Autodesk Fusion 360 part; units mm, degrees
(part 2 of 2)
sketch "Sketch3 (4)" plane through (0, 0, 356.35) normal (0, 0, 1) x (-1, 0, 0) in component "Roof"
  circle A0 centre (0, -130.225) radius 14.5
  line L0 (19.05, -257.175) -> (19.05, -263.525)
  line L1 (19.05, -263.525) -> (-19.05, -263.525)
  line L2 (-19.05, -263.525) -> (-19.05, -257.175)
  line L3 (-19.05, -257.175) -> (19.05, -257.175)
  line L4 (-126.35, -111.125) -> (-120, -111.125)
  line L5 (-120, -111.125) -> (-120, -149.225)
  line L6 (-120, -149.225) -> (-126.35, -149.225)
  line L7 (-126.35, -149.225) -> (-126.35, -111.125)
  line L8 (-19.05, 3.075) -> (19.05, 3.075)
  line L9 (19.05, 3.075) -> (19.05, -3.275)
  line L10 (19.05, -3.275) -> (-19.05, -3.275)
  line L11 (-19.05, -3.275) -> (-19.05, 3.075)
  line L12 (120, -111.1333) -> (126.35, -111.1333)
  line L13 (126.35, -111.1333) -> (126.35, -149.2333)
  line L14 (126.35, -149.2333) -> (120, -149.2333)
  line L15 (120, -149.2333) -> (120, -111.1333)
  line L16 (136.35, 13.325) -> (-136.35, 13.325)
  line L17 (-136.35, 13.325) -> (-136.35, -273.775)
  line L18 (-136.35, -273.775) -> (136.35, -273.775)
  line L19 (136.35, -273.775) -> (136.35, 13.325)
  circle A1 centre (0, -175.225) radius 10.5
  circle A2 centre (-14.1421, -189.3671) radius 6
  circle A3 centre (-14.1421, -161.0829) radius 6
  circle A4 centre (14.1421, -161.0829) radius 6
  circle A5 centre (14.1421, -189.3671) radius 6
  dimension "d238" = 21
  dimension "d239" = 12
  dimension "d240" = 12
  dimension "d241" = 12
  dimension "d242" = 12
  dimension "d243" = 20
  dimension "d244" = 20
  dimension "d245" = 20
  dimension "d246" = 20
  dimension "d247" = 45
  measures "d238" diameter of A1
  measures "d239" diameter of A2
  measures "d240" diameter of A3
  measures "d241" diameter of A4
  measures "d242" diameter of A5
  measures "d243" distance of A1.centre A4.centre
  measures "d244" distance of A1.centre A3.centre
  measures "d245" distance of A1.centre A2.centre
  measures "d246" distance of A1.centre A5.centre
  measures "d247" distance of A0.centre A1.centre
extrude "Extrude3'''" cut sketch "Sketch3 (4)" against normal blind 10 contours A1 | A2 | A3 | A4 | A5 bodies 9 in component "Roof"
sketch "Sketch4 (3)" plane through (0, 0, 356.35) normal (0, 0, 1) x (-1, 0, 0) in component "Roof"
  circle A0 centre (14.1421, -161.0829) radius 6
  circle A1 centre (0, -175.225) radius 10.5
  circle A2 centre (-14.1421, -161.0829) radius 6
  circle A3 centre (14.1421, -189.3671) radius 6
  circle A4 centre (-14.1421, -189.3671) radius 6
  circle A5 centre (0, -130.225) radius 14.5
  line L0 (19.05, -257.175) -> (19.05, -263.525)
  line L1 (19.05, -263.525) -> (-19.05, -263.525)
  line L2 (-19.05, -263.525) -> (-19.05, -257.175)
  line L3 (-19.05, -257.175) -> (19.05, -257.175)
  line L4 (-126.35, -111.125) -> (-120, -111.125)
  line L5 (-120, -111.125) -> (-120, -149.225)
  line L6 (-120, -149.225) -> (-126.35, -149.225)
  line L7 (-126.35, -149.225) -> (-126.35, -111.125)
  line L8 (-19.05, 3.075) -> (19.05, 3.075)
  line L9 (19.05, 3.075) -> (19.05, -3.275)
  line L10 (19.05, -3.275) -> (-19.05, -3.275)
  line L11 (-19.05, -3.275) -> (-19.05, 3.075)
  line L12 (120, -111.1333) -> (126.35, -111.1333)
  line L13 (126.35, -111.1333) -> (126.35, -149.2333)
  line L14 (126.35, -149.2333) -> (120, -149.2333)
  line L15 (120, -149.2333) -> (120, -111.1333)
  line L16 (136.35, 13.325) -> (-136.35, 13.325)
  line L17 (-136.35, 13.325) -> (-136.35, -273.775)
  line L18 (-136.35, -273.775) -> (136.35, -273.775)
  line L19 (136.35, -273.775) -> (136.35, 13.325)
  line L20 (-10.3078, -177.225) -> (-136.35, -177.225)
  line L21 (-136.35, -177.225) -> (-136.35, -173.225)
  line L22 (-136.35, -173.225) -> (-10.3078, -173.225)
  line L23 (-10.3078, -173.225) -> (-10.3078, -177.225)
  dimension "d250" = 2
  dimension "d251" = 2
  constraint horizontal L20
  constraint vertical L21
  constraint horizontal L22
  constraint vertical L23
  constraint coincident L17 L21.end
  constraint coincident A1 L20.start
  measures "d250" distance of A1.centre L20
  measures "d251" distance of A1.centre L22
extrude "Extrude4'''" cut sketch "Sketch4 (3)" against normal blind 6.35 contours A1 L17 L20 L21 L22 bodies 9 in component "Roof"
sketch "Sketch2 (5)" plane through (-126.35, 0, 0) normal (-1, 0, 0) x (0, -1, 0) in component "Left Wall"
  circle A0 centre (-130.175, 177.8) radius 31.75
  line L0 (-149.225, 25.4) -> (-149.225, 31.75)
  line L1 (-149.225, 31.75) -> (-111.125, 31.75)
  line L2 (-111.125, 31.75) -> (-111.125, 25.4)
  line L3 (-111.125, 25.4) -> (-149.225, 25.4)
  circle A1 centre (-183.675, 290) radius 5
  circle A2 centre (-98.075, 290) radius 5
  circle A3 centre (-33.875, 310) radius 5
  circle A4 centre (-119.475, 310) radius 5
  circle A5 centre (-205.075, 310) radius 5
  circle A6 centre (-183.675, 330) radius 5
  circle A7 centre (-98.075, 330) radius 5
  circle A8 centre (-33.875, 330) radius 5
  circle A9 centre (-119.475, 330) radius 5
  circle A10 centre (-205.075, 330) radius 5
  circle A11 centre (-183.675, 310) radius 5
  circle A12 centre (-98.075, 310) radius 5
  circle A13 centre (-33.875, 290) radius 5
  circle A14 centre (-119.475, 290) radius 5
  circle A15 centre (-205.075, 290) radius 5
  circle A16 centre (-162.275, 290) radius 5
  circle A17 centre (-76.675, 290) radius 5
  circle A18 centre (-55.275, 310) radius 5
  circle A19 centre (-162.275, 310) radius 5
  circle A20 centre (-226.4722, 310.344) radius 5
  circle A21 centre (-162.275, 330) radius 5
  circle A22 centre (-76.675, 330) radius 5
  circle A23 centre (-55.275, 330) radius 5
  circle A24 centre (-140.875, 330) radius 5
  circle A25 centre (-226.475, 330) radius 5
  circle A26 centre (-140.875, 310) radius 5
  circle A27 centre (-76.675, 310) radius 5
  circle A28 centre (-55.275, 290) radius 5
  circle A29 centre (-140.875, 290) radius 5
  circle A30 centre (-226.475, 290) radius 5
  line L4 (-3.175, 330.95) -> (-3.175, 350)
  line L5 (-3.175, 350) -> (-111.125, 350)
  line L6 (-111.125, 350) -> (-111.125, 370)
  line L7 (-111.125, 370) -> (-149.225, 370)
  line L8 (-149.225, 370) -> (-149.225, 350)
  line L9 (-149.225, 350) -> (-257.175, 350)
  line L10 (-257.175, 350) -> (-257.175, 330.95)
  line L11 (-257.175, 330.95) -> (-263.525, 330.95)
  line L12 (-263.525, 330.95) -> (-263.525, 350)
  line L13 (-263.525, 350) -> (-273.675, 350)
  line L14 (-273.675, 350) -> (-273.675, 311.9)
  line L15 (-273.675, 311.9) -> (-257.175, 311.9)
  line L16 (-257.175, 311.9) -> (-257.175, 0)
  line L17 (-257.175, 0) -> (-3.175, 0)
  line L18 (-3.175, 0) -> (-3.175, 311.9)
  line L19 (-3.175, 311.9) -> (13.325, 311.9)
  line L20 (13.325, 311.9) -> (13.325, 350)
  line L21 (13.325, 350) -> (3.175, 350)
  line L22 (3.175, 350) -> (3.175, 330.95)
  line L23 (3.175, 330.95) -> (-3.175, 330.95)
  line L24 (-140.175, 55.75) -> (-120.175, 55.75)
  line L25 (-120.175, 55.75) -> (-120.175, 43.75)
  line L26 (-120.175, 43.75) -> (-140.175, 43.75)
  line L27 (-140.175, 43.75) -> (-140.175, 55.75)
  dimension "d254" = 20
  dimension "d255" = 12
  dimension "d256" = 117
  dimension "d265" = 12
  constraint horizontal L24
  constraint vertical L25
  constraint horizontal L26
  constraint vertical L27
  measures "d254" distance of L24.start L24.end
  measures "d255" distance of L24.end L25.end
  measures "d256" distance of L18 L25
  measures "d265" distance of L1 L26
extrude "Extrude2'''''" cut sketch "Sketch2 (5)" against normal blind 20 contours L24 L25 L26 L27 bodies 6 in component "Left Wall"
sketch "Sketch1 (7)" plane through (0, -3.175, 0) normal (0, -1, 0) x (1, 0, 0) in component "Front Wall"
  line L0 (19.05, 31.75) -> (19.05, 25.4)
  line L1 (19.05, 25.4) -> (-19.05, 25.4)
  line L2 (-19.05, 25.4) -> (-19.05, 31.75)
  line L3 (-19.05, 31.75) -> (19.05, 31.75)
  circle A0 centre (50, 290) radius 5
  circle A1 centre (-30, 290) radius 5
  circle A2 centre (-90, 310) radius 5
  circle A3 centre (-10, 310) radius 5
  circle A4 centre (70, 310) radius 5
  circle A5 centre (50, 330) radius 5
  circle A6 centre (-30, 330) radius 5
  circle A7 centre (-90, 330) radius 5
  circle A8 centre (-10, 330) radius 5
  circle A9 centre (70, 330) radius 5
  circle A10 centre (50, 310) radius 5
  circle A11 centre (-30, 310) radius 5
  circle A12 centre (-90, 290) radius 5
  circle A13 centre (-10, 290) radius 5
  circle A14 centre (70, 290) radius 5
  circle A15 centre (30, 290) radius 5
  circle A16 centre (-50, 290) radius 5
  circle A17 centre (-70, 310) radius 5
  circle A18 centre (10, 310) radius 5
  circle A19 centre (90, 310) radius 5
  circle A20 centre (30, 330) radius 5
  circle A21 centre (-50, 330) radius 5
  circle A22 centre (-70, 330) radius 5
  circle A23 centre (10, 330) radius 5
  circle A24 centre (90, 330) radius 5
  circle A25 centre (30, 310) radius 5
  circle A26 centre (-50, 310) radius 5
  circle A27 centre (-70, 290) radius 5
  circle A28 centre (10, 290) radius 5
  circle A29 centre (90, 290) radius 5
  line L4 (-136.5, 350) -> (-136.5, 311.9)
  line L5 (-136.5, 311.9) -> (-126.35, 311.9)
  line L6 (-126.35, 311.9) -> (-126.35, 330.95)
  line L7 (-126.35, 330.95) -> (-120, 330.95)
  line L8 (-120, 330.95) -> (-120, 0)
  line L9 (-120, 0) -> (120, 0)
  line L10 (120, 0) -> (120, 330.95)
  line L11 (120, 330.95) -> (126.35, 330.95)
  line L12 (126.35, 330.95) -> (126.35, 311.9)
  line L13 (126.35, 311.9) -> (136.5, 311.9)
  line L14 (136.5, 311.9) -> (136.5, 350)
  line L15 (136.5, 350) -> (19.05, 350)
  line L16 (19.05, 350) -> (19.05, 370)
  line L17 (19.05, 370) -> (-19.05, 370)
  line L18 (-19.05, 370) -> (-19.05, 350)
  line L19 (-19.05, 350) -> (-136.5, 350)
  line L20 (-10, 55.75) -> (10, 55.75)
  line L21 (10, 55.75) -> (10, 43.75)
  line L22 (10, 43.75) -> (-10, 43.75)
  line L23 (-10, 43.75) -> (-10, 55.75)
  dimension "d259" = 12
  dimension "d260" = 20
  dimension "d261" = 10
  dimension "d264" = 12
  constraint horizontal L20
  constraint vertical L21
  constraint horizontal L22
  constraint vertical L23
  measures "d259" distance of L20.start L22.end
  measures "d260" distance of L20.start L20.end
  measures "d261" distance of origin L21
  measures "d264" distance of L3 L22
extrude "Extrude1''''''" cut sketch "Sketch1 (7)" against normal blind 20 contours L20 L21 L22 L23 bodies 7 in component "Front Wall"
sketch "Sketch9" plane through (126.35, 130.175, 185) normal (1, 0, 0) x (0, 1, 0) in component "Right wall"
  line L0 (-10, -129.25) -> (10, -129.25)
  line L1 (10, -129.25) -> (10, -141.25)
  line L2 (10, -141.25) -> (-10, -141.25)
  line L3 (-10, -141.25) -> (-10, -129.25)
  line L4 (-19.05, -153.25) -> (19.05, -153.25)
  dimension "d266" = 20
  dimension "d267" = 12
  dimension "d268" = 12
  constraint horizontal L0
  constraint vertical L1
  constraint horizontal L2
  constraint vertical L3
  measures "d266" distance of L0.start L0.end
  measures "d267" distance of L0.end L1.end
  measures "d268" distance of L2 L4
extrude "Extrude7" cut sketch "Sketch9" against normal blind 20 bodies 2 in component "Right wall"
component "Right wall" placed x (1, 0, 0) y (0, 1, 0) z (0, 0, 1) at (0, 0, 0)
component "Back Wall" placed x (1, 0, 0) y (0, 1, 0) z (0, 0, 1) at (0, 0, 0)
component "Left Wall" placed x (1, 0, 0) y (0, 1, 0) z (0, 0, 1) at (0, 0, 0)
component "Front Wall" placed x (1, 0, 0) y (0, 1, 0) z (0, 0, 1) at (0, 0, 0)
component "Floor" placed x (1, 0, 0) y (0, 1, 0) z (0, 0, 1) at (0, 0, 0)
component "Roof" placed x (1, 0, 0) y (0, 1, 0) z (0, 0, 1) at (0, 0, 0)
